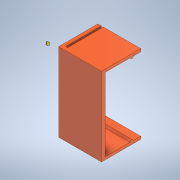
# Autodesk Inventor part: usbHubCaseTopPowerSide
Saved by Autodesk Inventor 2021.2 (Build 252289000, 289)
## iProperties
Created: 2021-02-17
Part Number: usbHubCaseTopPowerSide
Material: PC/ABS Plastic
Document SubType Name: Modeling
Designer: robst
Density: 0.357273 g/cm^3
Appearance: Smooth - Light Orange
Author: robst
Autodesk Inventor part; units mm, degrees
ref_plane "YZ Plane" through (0, 0, 0) normal (1, 0, 0) x (0, 1, 0)
ref_plane "XZ Plane" through (0, 0, 0) normal (0, 1, 0) x (-1, 0, 0)
ref_plane "XY Plane" through (0, 0, 0) normal (0, 0, 1) x (1, 0, 0)
sketch "Sketch1" plane through (0, 0, 0) normal (0, 0, 1) x (1, 0, 0)
  line L0 (-15.24, -27.94) -> (15.24, -27.94)
  line L1 (15.24, -27.94) -> (15.24, 27.94)
  line L2 (15.24, 27.94) -> (-15.24, 27.94)
  line L3 (-15.24, 27.94) -> (-15.24, -27.94)
  line L4 (-15.24, -27.94) -> (15.24, 27.94) construction
  line L5 (15.24, -27.94) -> (-15.24, 27.94) construction
  point P0 (0, 0)
  dimension "d0" = 55.88
  dimension "d1" = 30.48
  constraints: 12 end point, 2 midpoint, 2 parallel, 1 horizontal, 1 perpendicular
  measures "d0" distance of L2.end L0.start
  measures "d1" distance of L1.end L2.end
extrude "Extrusion1" add sketch "Sketch1" against normal blind 2.54
sketch "Sketch8" plane through (0, 0, -2.54) normal (0, 0, -1) x (-1, 0, 0)
  line L0 (-15.24, 27.94) -> (-15.24, -27.94) projected
  line L1 (15.24, -27.94) -> (15.24, 27.94) projected
  line L2 (-15.24, 27.94) -> (15.24, 27.94)
  line L3 (15.24, 27.94) -> (15.24, 26.035)
  line L4 (15.24, 26.035) -> (-15.24, 26.035)
  line L5 (-15.24, 26.035) -> (-15.24, 27.94)
  line L6 (-15.24, -27.94) -> (15.24, -27.94)
  line L7 (15.24, -27.94) -> (15.24, -26.035)
  line L8 (15.24, -26.035) -> (-15.24, -26.035)
  line L9 (-15.24, -26.035) -> (-15.24, -27.94)
  line L10 (15.24, 26.035) -> (12.7, 26.035)
  line L11 (12.7, 26.035) -> (12.7, 13.843)
  line L12 (12.7, 13.843) -> (15.24, 13.843)
  line L13 (15.24, 13.843) -> (15.24, 26.035)
  line L14 (15.24, -26.035) -> (12.7, -26.035)
  line L15 (12.7, -26.035) -> (12.7, -13.843)
  line L16 (12.7, -13.843) -> (15.24, -13.843)
  line L17 (15.24, -13.843) -> (15.24, -26.035)
  point P0 (0, 0)
  point P1 (15.24, -13.843)
  point P2 (-15.24, -26.035)
  dimension "d32" = 1.905
  dimension "d33" = 1.905
  dimension "d34" = 2.54
  dimension "d35" = 12.192
  dimension "d36" = 12.192
  dimension "d37" = 2.54
  constraints: 32 end point, 8 parallel, 4 horizontal, 4 perpendicular, 2 point on line
  measures "d32" distance between parallel lines of L4 L2
  measures "d33" distance between parallel lines of L8 L6
  measures "d34" distance between parallel lines of L11 L1
  measures "d35" distance between parallel lines of L12 L4
  measures "d36" distance between parallel lines of L16 L8
  measures "d37" distance between parallel lines of L1 L15
extrude "Extrusion7" add sketch "Sketch8" along normal blind 25.4 contours L2 L1 L4 L0 | L8 L1 L6 L0 | L4 L1 L12 L11 | L15 L16 L1 L8
sketch "Sketch10" plane through (0, 0, -2.54) normal (0, 0, -1) x (-1, 0, 0)
  line L0 (12.7, 26.035) -> (12.7, 13.843) projected
  line L1 (12.7, 13.843) -> (15.24, 13.843)
  line L2 (15.24, 13.843) -> (15.24, -13.843)
  line L3 (15.24, -13.843) -> (12.7, -13.843)
  line L4 (12.7, -13.843) -> (12.7, 13.843)
  point P0 (0, 0)
  constraints: 8 end point, 2 parallel, 1 horizontal, 1 perpendicular
extrude "Extrusion8" add sketch "Sketch10" along normal blind 6.096
sketch "Sketch11" plane through (15.24, -27.94, 0) normal (1, 0, 0) x (0, 0, -1)
  line L0 (2.54, 1.905) -> (27.94, 1.905) projected
  line L1 (2.54, 53.975) -> (27.94, 53.975) projected
  line L2 (20.32, 1.905) -> (21.59, 3.175)
  line L3 (21.59, 3.175) -> (22.86, 1.905)
  line L4 (2.54, 1.905) -> (27.94, 1.905) projected
  line L5 (27.94, 14.097) -> (27.94, 1.905) projected
  line L6 (20.32, 1.905) -> (22.86, 1.905)
  line L7 (0, 27.94) -> (27.94, 27.94) construction
  line L8 (2.54, 53.975) -> (27.94, 53.975)
  line L9 (20.32, 53.975) -> (21.59, 52.705)
  line L10 (21.59, 52.705) -> (22.86, 53.975)
  point P0 (22.86, 53.975)
  point P1 (22.86, 1.905)
  dimension "d42" = 90
  dimension "d43" = 135
  dimension "d44" = 1.27
  dimension "d45" = 6.35
  constraints: 14 end point, 3 point on line, 3 symmetric about line, 1 collinear, 1 horizontal
  measures "d42" angle of L3 L2
  measures "d43" angle of L3 L0
  measures "d44" distance from line of L2.end L0
  measures "d45" distance from line of L2.end L5
extrude "Extrusion9" add sketch "Sketch11" against normal up to surface (27.94 mm away)
sketch "Sketch12" plane through (-15.24, 27.94, 0) normal (0, 1, 0) x (1, 0, 0)
  line L0 (2.54, 2.54) -> (2.54, 20.32) projected
  line L1 (2.54, 22.86) -> (2.54, 27.94) projected
  line L2 (2.54, 27.94) -> (3.81, 27.94)
  line L3 (3.81, 27.94) -> (3.81, 2.54)
  line L4 (3.81, 2.54) -> (2.54, 2.54)
  line L5 (2.54, 2.54) -> (2.54, 27.94)
  point P0 (15.24, 0)
  point P1 (2.54, 22.86)
  point P2 (2.54, 20.32)
  dimension "d48" = 1.27
  constraints: 8 end point, 2 parallel, 1 horizontal, 1 perpendicular
  measures "d48" distance between parallel lines of L1 L3
extrude "Extrusion10" cut sketch "Sketch12" against normal through all
sketch "Sketch13" plane through (0, 0, -2.54) normal (0, 0, -1) x (-1, 0, 0)
  line L0 (-15.24, 27.94) -> (15.24, 27.94) construction
  line L1 (-1.27, 27.94) -> (-1.27, -28.2825) construction
  line L2 (-15.24, 26.035) -> (-15.24, -26.035) construction
  spline S0 degree 2 poles (-5.2014, -4.1958) (-4.9544, -4.1958) (-4.5098, -4.3718) (-4.3555, -4.5293) knots 0 0 0 1 2 2 2
  spline S1 degree 2 poles (-4.3555, -4.5293) (-4.1609, -4.7269) (-3.9603, -5.261) (-3.9603, -5.6686) knots 0 0 0 1 2 2 2
  line L3 (-3.9603, -5.6686) -> (-3.9603, -6.0978)
  line L4 (-3.9603, -6.0978) -> (-2.54, -6.0978)
  line L5 (-2.54, -6.0978) -> (-2.54, -6.6041)
  line L6 (-2.54, -6.6041) -> (-6.35, -6.6041)
  line L7 (-6.35, -6.6041) -> (-6.35, -5.647)
  spline S2 degree 2 poles (-6.35, -5.647) (-6.35, -5.3073) (-6.2388, -4.8319) (-6.1123, -4.6497) knots 0 0 0 1 2 2 2
  spline S3 degree 2 poles (-6.1123, -4.6497) (-5.9671, -4.4367) (-5.5195, -4.1958) (-5.2014, -4.1958) knots 0 0 0 1 2 2 2
  spline S4 degree 2 poles (-5.186, -4.7238) (-5.3836, -4.7238) (-5.6738, -4.8597) (-5.7665, -4.9986) knots 0 0 0 1 2 2 2
  spline S5 degree 2 poles (-5.7665, -4.9986) (-5.8467, -5.119) (-5.9116, -5.4401) (-5.9116, -5.6778) knots 0 0 0 1 2 2 2
  line L8 (-5.9116, -5.6778) -> (-5.9116, -6.0978)
  line L9 (-5.9116, -6.0978) -> (-4.3925, -6.0978)
  line L10 (-4.3925, -6.0978) -> (-4.3925, -5.7519)
  spline S6 degree 2 poles (-4.3925, -5.7519) (-4.3925, -5.4432) (-4.4913, -5.0634) (-4.621, -4.9399) knots 0 0 0 1 2 2 2
  spline S7 degree 2 poles (-4.621, -4.9399) (-4.7352, -4.8257) (-5.0038, -4.7238) (-5.186, -4.7238) knots 0 0 0 1 2 2 2
  line L11 (-6.35, -0.9509) -> (-2.54, -2.263)
  line L12 (-2.54, -2.263) -> (-2.54, -2.8095)
  line L13 (-2.54, -2.8095) -> (-6.35, -4.1217)
  line L14 (-6.35, -4.1217) -> (-6.35, -3.5783)
  line L15 (-6.35, -3.5783) -> (-3.1853, -2.5224)
  line L16 (-3.1853, -2.5224) -> (-6.35, -1.4665)
  line L17 (-6.35, -1.4665) -> (-6.35, -0.9509)
  line L18 (-3.9757, 0.7442) -> (-3.9757, -0.6977)
  line L19 (-3.9757, -0.6977) -> (-4.4388, -0.6977)
  line L20 (-4.4388, -0.6977) -> (-4.4388, 0.7442)
  line L21 (-4.4388, 0.7442) -> (-3.9757, 0.7442)
  spline S8 degree 2 poles (-4.445, 3.6218) (-3.4199, 3.6218) (-2.4597, 3.0259) (-2.4597, 2.4053) knots 0 0 0 1 2 2 2
  spline S9 degree 2 poles (-2.4597, 2.4053) (-2.4597, 1.7754) (-3.4385, 1.1857) (-4.4419, 1.1857) knots 0 0 0 1 2 2 2
  spline S10 degree 2 poles (-4.4419, 1.1857) (-5.4731, 1.1857) (-6.4272, 1.7816) (-6.4272, 2.4053) knots 0 0 0 1 2 2 2
  spline S11 degree 2 poles (-6.4272, 2.4053) (-6.4272, 3.032) (-5.4392, 3.6218) (-4.445, 3.6218) knots 0 0 0 1 2 2 2
  spline S12 degree 2 poles (-3.2841, 2.9672) (-3.4724, 3.0413) (-4.0529, 3.1031) (-4.445, 3.1031) knots 0 0 0 1 2 2 2
  spline S13 degree 2 poles (-4.445, 3.1031) (-4.8371, 3.1031) (-5.4145, 3.0413) (-5.609, 2.9641) knots 0 0 0 1 2 2 2
  spline S14 degree 2 poles (-5.609, 2.9641) (-5.8035, 2.8869) (-6.0042, 2.6183) (-6.0042, 2.4053) knots 0 0 0 1 2 2 2
  spline S15 degree 2 poles (-6.0042, 2.4053) (-6.0042, 2.1922) (-5.8035, 1.9175) (-5.6028, 1.8372) knots 0 0 0 1 2 2 2
  spline S16 degree 2 poles (-5.6028, 1.8372) (-5.4083, 1.76) (-4.8155, 1.7044) (-4.4419, 1.7044) knots 0 0 0 1 2 2 2
  spline S17 degree 2 poles (-4.4419, 1.7044) (-4.0405, 1.7044) (-3.5033, 1.7538) (-3.2934, 1.8341) knots 0 0 0 1 2 2 2
  spline S18 degree 2 poles (-3.2934, 1.8341) (-3.0958, 1.9082) (-2.8827, 2.183) (-2.8827, 2.4053) knots 0 0 0 1 2 2 2
  spline S19 degree 2 poles (-2.8827, 2.4053) (-2.8827, 2.6152) (-3.0834, 2.89) (-3.2841, 2.9672) knots 0 0 0 1 2 2 2
  line L22 (-2.54, 6.4592) -> (-2.54, 4.1096)
  line L23 (-2.54, 4.1096) -> (-3.0803, 4.1096)
  spline S20 degree 2 poles (-3.0803, 4.1096) (-3.3181, 4.3628) (-3.7596, 4.8135) (-3.9973, 5.0297) knots 0 0 0 1 2 2 2
  spline S21 degree 2 poles (-3.9973, 5.0297) (-4.4759, 5.465) (-5.0502, 5.783) (-5.3558, 5.783) knots 0 0 0 1 2 2 2
  spline S22 degree 2 poles (-5.3558, 5.783) (-5.5164, 5.783) (-5.7572, 5.6842) (-5.8344, 5.5947) knots 0 0 0 1 2 2 2
  spline S23 degree 2 poles (-5.8344, 5.5947) (-5.9116, 5.5052) (-5.9888, 5.2705) (-5.9888, 5.1285) knots 0 0 0 1 2 2 2
  spline S24 degree 2 poles (-5.9888, 5.1285) (-5.9888, 4.9926) (-5.9208, 4.7147) (-5.8683, 4.5882) knots 0 0 0 1 2 2 2
  spline S25 degree 2 poles (-5.8683, 4.5882) (-5.8251, 4.4801) (-5.7016, 4.2794) (-5.6584, 4.2177) knots 0 0 0 1 2 2 2
  line L24 (-5.6584, 4.2177) -> (-5.6584, 4.1899)
  line L25 (-5.6584, 4.1899) -> (-6.2018, 4.1899)
  spline S26 degree 2 poles (-6.2018, 4.1899) (-6.279, 4.3473) (-6.4303, 4.9123) (-6.4303, 5.1655) knots 0 0 0 1 2 2 2
  spline S27 degree 2 poles (-6.4303, 5.1655) (-6.4303, 5.6997) (-5.8653, 6.3017) (-5.3836, 6.3017) knots 0 0 0 1 2 2 2
  spline S28 degree 2 poles (-5.3836, 6.3017) (-5.1582, 6.3017) (-4.7815, 6.1968) (-4.621, 6.1041) knots 0 0 0 1 2 2 2
  spline S29 degree 2 poles (-4.621, 6.1041) (-4.4543, 6.0115) (-4.127, 5.7429) (-3.9695, 5.5947) knots 0 0 0 1 2 2 2
  spline S30 degree 2 poles (-3.9695, 5.5947) (-3.7071, 5.3539) (-3.1452, 4.7641) (-2.9815, 4.5882) knots 0 0 0 1 2 2 2
  line L26 (-2.9815, 4.5882) -> (-2.9815, 6.4592)
  line L27 (-2.9815, 6.4592) -> (-2.54, 6.4592)
  spline S31 degree 2 poles (1.1798, -10.2134) (1.4268, -10.2134) (1.8714, -10.3894) (2.0258, -10.5469) knots 0 0 0 1 2 2 2
  spline S32 degree 2 poles (2.0258, -10.5469) (2.2203, -10.7445) (2.421, -11.2786) (2.421, -11.6862) knots 0 0 0 1 2 2 2
  line L28 (2.421, -11.6862) -> (2.421, -12.1153)
  line L29 (2.421, -12.1153) -> (3.8412, -12.1153)
  line L30 (3.8412, -12.1153) -> (3.8412, -12.6217)
  line L31 (3.8412, -12.6217) -> (0.0312, -12.6217)
  line L32 (0.0312, -12.6217) -> (0.0312, -11.6645)
  spline S33 degree 2 poles (0.0312, -11.6645) (0.0312, -11.3249) (0.1424, -10.8494) (0.269, -10.6673) knots 0 0 0 1 2 2 2
  spline S34 degree 2 poles (0.269, -10.6673) (0.4141, -10.4542) (0.8618, -10.2134) (1.1798, -10.2134) knots 0 0 0 1 2 2 2
  spline S35 degree 2 poles (1.1952, -10.7414) (0.9976, -10.7414) (0.7074, -10.8772) (0.6148, -11.0162) knots 0 0 0 1 2 2 2
  spline S36 degree 2 poles (0.6148, -11.0162) (0.5345, -11.1366) (0.4696, -11.4577) (0.4696, -11.6954) knots 0 0 0 1 2 2 2
  line L33 (0.4696, -11.6954) -> (0.4696, -12.1153)
  line L34 (0.4696, -12.1153) -> (1.9887, -12.1153)
  line L35 (1.9887, -12.1153) -> (1.9887, -11.7695)
  spline S37 degree 2 poles (1.9887, -11.7695) (1.9887, -11.4608) (1.8899, -11.081) (1.7602, -10.9575) knots 0 0 0 1 2 2 2
  spline S38 degree 2 poles (1.7602, -10.9575) (1.646, -10.8433) (1.3774, -10.7414) (1.1952, -10.7414) knots 0 0 0 1 2 2 2
  spline S39 degree 2 poles (2.4117, -7.4192) (3.1342, -7.4192) (3.9215, -8.1139) (3.9215, -8.6944) knots 0 0 0 1 2 2 2
  spline S40 degree 2 poles (3.9215, -8.6944) (3.9215, -9.2902) (3.1095, -9.9726) (2.4117, -9.9726) knots 0 0 0 1 2 2 2
  spline S41 degree 2 poles (2.4117, -9.9726) (1.6954, -9.9726) (0.9019, -9.2686) (0.9019, -8.6944) knots 0 0 0 1 2 2 2
  spline S42 degree 2 poles (0.9019, -8.6944) (0.9019, -8.1139) (1.6923, -7.4192) (2.4117, -7.4192) knots 0 0 0 1 2 2 2
  spline S43 degree 2 poles (2.4117, -7.9163) (1.8559, -7.9163) (1.3156, -8.3208) (1.3156, -8.6944) knots 0 0 0 1 2 2 2
  spline S44 degree 2 poles (1.3156, -8.6944) (1.3156, -9.0679) (1.8559, -9.4755) (2.4117, -9.4755) knots 0 0 0 1 2 2 2
  spline S45 degree 2 poles (2.4117, -9.4755) (2.952, -9.4755) (3.5078, -9.0679) (3.5078, -8.6944) knots 0 0 0 1 2 2 2
  spline S46 degree 2 poles (3.5078, -8.6944) (3.5078, -8.3239) (2.9613, -7.9163) (2.4117, -7.9163) knots 0 0 0 1 2 2 2
  line L36 (0.9822, -3.461) -> (3.8412, -4.1866)
  line L37 (3.8412, -4.1866) -> (3.8412, -4.6312)
  line L38 (3.8412, -4.6312) -> (1.6367, -5.329)
  line L39 (1.6367, -5.329) -> (3.8412, -6.0236)
  line L40 (3.8412, -6.0236) -> (3.8412, -6.4652)
  line L41 (3.8412, -6.4652) -> (0.9822, -7.1969)
  line L42 (0.9822, -7.1969) -> (0.9822, -6.6967)
  line L43 (0.9822, -6.6967) -> (3.1959, -6.1904)
  line L44 (3.1959, -6.1904) -> (0.9822, -5.5142)
  line L45 (0.9822, -5.5142) -> (0.9822, -5.1159)
  line L46 (0.9822, -5.1159) -> (3.1959, -4.4212)
  line L47 (3.1959, -4.4212) -> (0.9822, -3.9457)
  line L48 (0.9822, -3.9457) -> (0.9822, -3.461)
  spline S47 degree 2 poles (3.9061, -1.7968) (3.9061, -2.4823) (3.1373, -3.2356) (2.4271, -3.2356) knots 0 0 0 1 2 2 2
  spline S48 degree 2 poles (2.4271, -3.2356) (1.7294, -3.2356) (0.9019, -2.5039) (0.9019, -1.9142) knots 0 0 0 1 2 2 2
  spline S49 degree 2 poles (0.9019, -1.9142) (0.9019, -1.6486) (1.0563, -1.238) (1.2199, -1.0867) knots 0 0 0 1 2 2 2
  spline S50 degree 2 poles (1.2199, -1.0867) (1.3836, -0.9323) (1.8559, -0.7687) (2.1987, -0.7687) knots 0 0 0 1 2 2 2
  line L49 (2.1987, -0.7687) -> (2.4611, -0.7687)
  line L50 (2.4611, -0.7687) -> (2.4611, -2.7478)
  spline S51 degree 2 poles (2.4611, -2.7478) (2.9582, -2.7478) (3.4862, -2.2476) (3.4862, -1.803) knots 0 0 0 1 2 2 2
  spline S52 degree 2 poles (3.4862, -1.803) (3.4862, -1.6455) (3.4151, -1.3399) (3.3596, -1.2164) knots 0 0 0 1 2 2 2
  spline S53 degree 2 poles (3.3596, -1.2164) (3.2978, -1.0867) (3.1898, -0.9076) (3.1403, -0.849) knots 0 0 0 1 2 2 2
  line L51 (3.1403, -0.849) -> (3.1403, -0.8212)
  line L52 (3.1403, -0.8212) -> (3.6652, -0.8212)
  spline S54 degree 2 poles (3.6652, -0.8212) (3.6992, -0.9045) (3.798, -1.1577) (3.8258, -1.2565) knots 0 0 0 1 2 2 2
  spline S55 degree 2 poles (3.8258, -1.2565) (3.8659, -1.3955) (3.9061, -1.6239) (3.9061, -1.7968) knots 0 0 0 1 2 2 2
  spline S56 degree 2 poles (2.0937, -1.238) (1.8992, -1.2442) (1.6151, -1.3244) (1.5194, -1.4016) knots 0 0 0 1 2 2 2
  spline S57 degree 2 poles (1.5194, -1.4016) (1.4113, -1.485) (1.2971, -1.7474) (1.2971, -1.9419) knots 0 0 0 1 2 2 2
  spline S58 degree 2 poles (1.2971, -1.9419) (1.2971, -2.1334) (1.4113, -2.402) (1.5225, -2.5131) knots 0 0 0 1 2 2 2
  spline S59 degree 2 poles (1.5225, -2.5131) (1.6367, -2.6212) (1.9115, -2.7324) (2.0937, -2.7478) knots 0 0 0 1 2 2 2
  line L53 (2.0937, -2.7478) -> (2.0937, -1.238)
  line L54 (1.4978, 1.2351) -> (1.4978, 1.2104)
  spline S60 degree 2 poles (1.4978, 1.2104) (1.4824, 1.1548) (1.4762, 1.0344) (1.4762, 0.9511) knots 0 0 0 1 2 2 2
  spline S61 degree 2 poles (1.4762, 0.9511) (1.4762, 0.7565) (1.646, 0.3737) (1.8127, 0.2008) knots 0 0 0 1 2 2 2
  line L55 (1.8127, 0.2008) -> (3.8412, 0.2008)
  line L56 (3.8412, 0.2008) -> (3.8412, -0.2809)
  line L57 (3.8412, -0.2809) -> (0.9822, -0.2809)
  line L58 (0.9822, -0.2809) -> (0.9822, 0.2008)
  line L59 (0.9822, 0.2008) -> (1.4083, 0.2008)
  spline S62 degree 2 poles (1.4083, 0.2008) (1.1736, 0.4632) (0.9822, 0.8553) (0.9822, 1.0406) knots 0 0 0 1 2 2 2
  spline S63 degree 2 poles (0.9822, 1.0406) (0.9822, 1.1147) (0.9883, 1.1888) (0.9976, 1.2351) knots 0 0 0 1 2 2 2
  line L60 (0.9976, 1.2351) -> (1.4978, 1.2351)
  spline S64 degree 2 poles (3.9091, 4.3442) (3.9091, 3.9305) (3.7362, 3.3501) (3.6127, 3.0938) knots 0 0 0 1 2 2 2
  line L61 (3.6127, 3.0938) -> (2.9767, 3.0938)
  line L62 (2.9767, 3.0938) -> (2.9767, 3.1308)
  spline S65 degree 2 poles (2.9767, 3.1308) (3.2114, 3.3809) (3.4707, 4.0139) (3.4707, 4.3072) knots 0 0 0 1 2 2 2
  spline S66 degree 2 poles (3.4707, 4.3072) (3.4707, 4.7271) (3.1218, 5.1563) (2.8347, 5.1563) knots 0 0 0 1 2 2 2
  spline S67 degree 2 poles (2.8347, 5.1563) (2.6062, 5.1563) (2.3222, 4.9309) (2.2511, 4.687) knots 0 0 0 1 2 2 2
  spline S68 degree 2 poles (2.2511, 4.687) (2.2017, 4.511) (2.1338, 4.2177) (2.0782, 3.9984) knots 0 0 0 1 2 2 2
  spline S69 degree 2 poles (2.0782, 3.9984) (2.0258, 3.8008) (1.8683, 3.489) (1.7417, 3.3686) knots 0 0 0 1 2 2 2
  spline S70 degree 2 poles (1.7417, 3.3686) (1.6151, 3.2513) (1.2755, 3.1216) (1.0532, 3.1216) knots 0 0 0 1 2 2 2
  spline S71 degree 2 poles (1.0532, 3.1216) (0.5901, 3.1216) (-0.0367, 3.8441) (-0.0367, 4.4029) knots 0 0 0 1 2 2 2
  spline S72 degree 2 poles (-0.0367, 4.4029) (-0.0367, 4.724) (0.0899, 5.2921) (0.2103, 5.536) knots 0 0 0 1 2 2 2
  line L63 (0.2103, 5.536) -> (0.8154, 5.536)
  line L64 (0.8154, 5.536) -> (0.8154, 5.499)
  spline S73 degree 2 poles (0.8154, 5.499) (0.6487, 5.3168) (0.4017, 4.7487) (0.4017, 4.4369) knots 0 0 0 1 2 2 2
  spline S74 degree 2 poles (0.4017, 4.4369) (0.4017, 4.0849) (0.7321, 3.6496) (1.0007, 3.6496) knots 0 0 0 1 2 2 2
  spline S75 degree 2 poles (1.0007, 3.6496) (1.2415, 3.6496) (1.5287, 3.9058) (1.5935, 4.1466) knots 0 0 0 1 2 2 2
  spline S76 degree 2 poles (1.5935, 4.1466) (1.6367, 4.3072) (1.7479, 4.7734) (1.7942, 4.9278) knots 0 0 0 1 2 2 2
  spline S77 degree 2 poles (1.7942, 4.9278) (1.9146, 5.3199) (2.3993, 5.6842) (2.7544, 5.6842) knots 0 0 0 1 2 2 2
  spline S78 degree 2 poles (2.7544, 5.6842) (2.9798, 5.6842) (3.4121, 5.5021) (3.5633, 5.3384) knots 0 0 0 1 2 2 2
  spline S79 degree 2 poles (3.5633, 5.3384) (3.7301, 5.1563) (3.9091, 4.6931) (3.9091, 4.3442) knots 0 0 0 1 2 2 2
  line L65 (3.8412, 6.6537) -> (3.8412, 6.1721)
  line L66 (3.8412, 6.1721) -> (0.9822, 6.1721)
  line L67 (0.9822, 6.1721) -> (0.9822, 6.6537)
  line L68 (0.9822, 6.6537) -> (3.8412, 6.6537)
  line L69 (0.5067, 6.6877) -> (0.5067, 6.1412)
  line L70 (0.5067, 6.1412) -> (0.0065, 6.1412)
  line L71 (0.0065, 6.1412) -> (0.0065, 6.6877)
  line L72 (0.0065, 6.6877) -> (0.5067, 6.6877)
  line L73 (3.8412, 9.5591) -> (3.8412, 9.0774)
  line L74 (3.8412, 9.0774) -> (3.551, 9.0774)
  spline S80 degree 2 poles (3.551, 9.0774) (3.6436, 8.9663) (3.7671, 8.8026) (3.8196, 8.6915) knots 0 0 0 1 2 2 2
  spline S81 degree 2 poles (3.8196, 8.6915) (3.869, 8.5896) (3.9215, 8.3704) (3.9215, 8.2253) knots 0 0 0 1 2 2 2
  spline S82 degree 2 poles (3.9215, 8.2253) (3.9215, 7.9906) (3.727, 7.5954) (3.5386, 7.4565) knots 0 0 0 1 2 2 2
  spline S83 degree 2 poles (3.5386, 7.4565) (3.3503, 7.3175) (2.7945, 7.1631) (2.4333, 7.1631) knots 0 0 0 1 2 2 2
  spline S84 degree 2 poles (2.4333, 7.1631) (2.0566, 7.1631) (1.5071, 7.3577) (1.3002, 7.5275) knots 0 0 0 1 2 2 2
  spline S85 degree 2 poles (1.3002, 7.5275) (1.1149, 7.6849) (0.9019, 8.1265) (0.9019, 8.3704) knots 0 0 0 1 2 2 2
  spline S86 degree 2 poles (0.9019, 8.3704) (0.9019, 8.5834) (0.9976, 8.9014) (1.0964, 9.0774) knots 0 0 0 1 2 2 2
  line L75 (1.0964, 9.0774) -> (-0.1386, 9.0774)
  line L76 (-0.1386, 9.0774) -> (-0.1386, 9.5591)
  line L77 (-0.1386, 9.5591) -> (3.8412, 9.5591)
  line L78 (3.1465, 9.0774) -> (1.4947, 9.0774)
  spline S87 degree 2 poles (1.4947, 9.0774) (1.4083, 8.8983) (1.3434, 8.6143) (1.3434, 8.4506) knots 0 0 0 1 2 2 2
  spline S88 degree 2 poles (1.3434, 8.4506) (1.3434, 8.0801) (1.8992, 7.6602) (2.424, 7.6602) knots 0 0 0 1 2 2 2
  spline S89 degree 2 poles (2.424, 7.6602) (2.9304, 7.6602) (3.4645, 7.9813) (3.4645, 8.3364) knots 0 0 0 1 2 2 2
  spline S90 degree 2 poles (3.4645, 8.3364) (3.4645, 8.5247) (3.2916, 8.9076) (3.1465, 9.0774) knots 0 0 0 1 2 2 2
  spline S91 degree 2 poles (3.9061, 11.498) (3.9061, 10.8126) (3.1373, 10.0592) (2.4271, 10.0592) knots 0 0 0 1 2 2 2
  spline S92 degree 2 poles (2.4271, 10.0592) (1.7294, 10.0592) (0.9019, 10.791) (0.9019, 11.3807) knots 0 0 0 1 2 2 2
  spline S93 degree 2 poles (0.9019, 11.3807) (0.9019, 11.6462) (1.0563, 12.0569) (1.2199, 12.2082) knots 0 0 0 1 2 2 2
  spline S94 degree 2 poles (1.2199, 12.2082) (1.3836, 12.3625) (1.8559, 12.5262) (2.1987, 12.5262) knots 0 0 0 1 2 2 2
  line L79 (2.1987, 12.5262) -> (2.4611, 12.5262)
  line L80 (2.4611, 12.5262) -> (2.4611, 10.5471)
  spline S95 degree 2 poles (2.4611, 10.5471) (2.9582, 10.5471) (3.4862, 11.0473) (3.4862, 11.4919) knots 0 0 0 1 2 2 2
  spline S96 degree 2 poles (3.4862, 11.4919) (3.4862, 11.6493) (3.4151, 11.955) (3.3596, 12.0785) knots 0 0 0 1 2 2 2
  spline S97 degree 2 poles (3.3596, 12.0785) (3.2978, 12.2082) (3.1898, 12.3872) (3.1403, 12.4459) knots 0 0 0 1 2 2 2
  line L81 (3.1403, 12.4459) -> (3.1403, 12.4737)
  line L82 (3.1403, 12.4737) -> (3.6652, 12.4737)
  spline S98 degree 2 poles (3.6652, 12.4737) (3.6992, 12.3903) (3.798, 12.1371) (3.8258, 12.0383) knots 0 0 0 1 2 2 2
  spline S99 degree 2 poles (3.8258, 12.0383) (3.8659, 11.8994) (3.9061, 11.6709) (3.9061, 11.498) knots 0 0 0 1 2 2 2
  spline S100 degree 2 poles (2.0937, 12.0569) (1.8992, 12.0507) (1.6151, 11.9704) (1.5194, 11.8932) knots 0 0 0 1 2 2 2
  spline S101 degree 2 poles (1.5194, 11.8932) (1.4113, 11.8099) (1.2971, 11.5474) (1.2971, 11.3529) knots 0 0 0 1 2 2 2
  spline S102 degree 2 poles (1.2971, 11.3529) (1.2971, 11.1615) (1.4113, 10.8929) (1.5225, 10.7817) knots 0 0 0 1 2 2 2
  spline S103 degree 2 poles (1.5225, 10.7817) (1.6367, 10.6737) (1.9115, 10.5625) (2.0937, 10.5471) knots 0 0 0 1 2 2 2
  line L83 (2.0937, 10.5471) -> (2.0937, 12.0569)
  point P0 (0, 0)
  dimension "d51" = 13.97
  constraints: 2 end point, 2 vertical, 1 point on line
  measures "d51" distance between parallel lines of L1 L2
extrude "Extrusion11" cut sketch "Sketch13" against normal blind 1.27
equation "\"d2\" = usbHolderWallThickness"
equation "\"usbHolderWallThickness\" = 2.54"
equation "\"usbHubWidth\" = 44.45"
equation "\"usbHubDepth\" = 27.432"
equation "\"usbHubLength\" = 109.22"
equation "\"usbHolderWidth\" = 58.42"
equation "\"usbHolderLength\" = usbHubLength + 2 * usbHolderWallThickness"
equation "\"holePatternLength\" = 25.4"
equation "\"holePatternWidth\" = 50.8"
body "Solid1"
